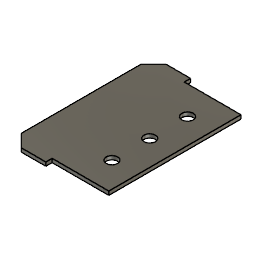
GPL H250 to H250G9 (Autodesk Fusion 360 design; units mm, degrees)
Autodesk Fusion 360 part; units mm, degrees
sketch "スケッチ1" plane through (0, 0, 0) normal (0, 0, 1) x (1, 0, 0)
  line L0 (-15.5, 115) -> (-74.5, 115)
  line L1 (-74.5, 115) -> (-74.5, -115)
  line L2 (-74.5, -115) -> (-15.5, -115)
  line L3 (74.5, -105) -> (74.5, 105)
  line L4 (68.0217, 105) -> (-74.5, -115) construction
  line L5 (-74.5, 115) -> (68.0217, -105) construction
  line L6 (-15.5, 115) -> (-15.5, 105)
  line L7 (-15.5, 105) -> (74.5, 105)
  line L8 (-15.5, -115) -> (-15.5, -105)
  line L9 (-15.5, -105) -> (74.5, -105)
  dimension "d2" = 230
  constraint horizontal L0
  constraint perpendicular L0 L1
  constraint parallel L0 L2
  constraint parallel L1 L3
  constraint coincident L4 origin
  constraint coincident L5 origin
  constraint vertical L6
  constraint horizontal L7
  constraint coincident L7 L4.start
  constraint vertical L8
  constraint horizontal L9
  constraint coincident L9 L5.end
  measures "d2" distance of L0.end L1.end
extrude "押し出し1" add sketch "スケッチ1" along normal blind 6
chamfer "面取り1" distance 20 angle 45 2 edges at (-74.5, -115, 3) (-74.5, 115, 3)
sketch "スケッチ2" plane through (0, 0, 6) normal (0, 0, 1) x (-1, 0, 0)
  line L0 (54.5, -115) -> (74.5, -95)
  line L1 (74.5, -95) -> (74.5, 95)
  line L2 (74.5, 95) -> (54.5, 115)
  line L3 (54.5, 115) -> (15.5, 115)
  line L4 (15.5, 115) -> (15.5, 105)
  line L5 (15.5, 105) -> (-74.5, 105)
  line L6 (-74.5, 105) -> (-74.5, -105)
  line L7 (-74.5, -105) -> (15.5, -105)
  line L8 (15.5, -105) -> (15.5, -115)
  line L9 (15.5, -115) -> (54.5, -115)
  line L10 (-74.5, -105) -> (-34.5, -105)
  line L11 (-34.5, -105) -> (-34.5, -60)
  line L12 (-34.5, -60) -> (-74.5, -60)
  line L13 (-74.5, -60) -> (-74.5, -105)
  line L14 (-34.5, -60) -> (-34.5, 0)
  line L15 (-34.5, 0) -> (-34.5, 60)
  point P0 (-34.5, -60)
  point P1 (-34.5, 0)
  point P2 (-34.5, 60)
  dimension "d10" = 40
  dimension "d11" = 45
  dimension "d12" = 60
  dimension "d13" = 60
  constraint horizontal L10
  constraint vertical L11
  constraint horizontal L12
  constraint vertical L13
  constraint coincident L6.end L7.start
  constraint perpendicular L12 L14
  constraint parallel L14 L15
  constraint coincident P0 L11.end
  constraint coincident P1 L14.end
  constraint coincident P2 L15.end
  measures "d10" distance of L6.end L10.end
  measures "d11" distance of L6.end L12.end
  measures "d12" distance of P0 P1
  measures "d13" distance of P1 P2
hole "穴1" at (34.5, 60, 6) at (34.5, 0, 6) at (34.5, -60, 6) direction (0, 0, -1) diameter 18 end through all
